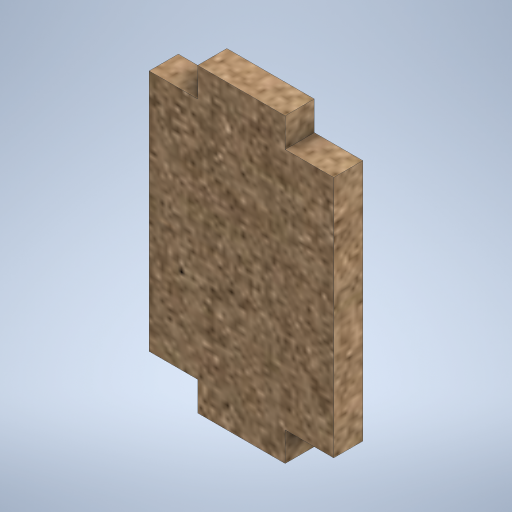
# Autodesk Inventor part: Wall_Base2
Saved by Autodesk Inventor 2024 (Build 280153000, 153)
## iProperties
Created: 2023-11-23
Part Number: Wall_Base2
Material: MDF Tablero de fibras de densidad media
Document SubType Name: Modeling
Designer: marco
Density: 0.8 g/cm^3
Appearance: Cartón - Ondulado
Author: marco
Autodesk Inventor part; units mm, degrees
ref_plane "YZ Plane" through (0, 0, 0) normal (1, 0, 0) x (0, 1, 0)
ref_plane "XZ Plane" through (0, 0, 0) normal (0, 1, 0) x (-1, 0, 0)
ref_plane "XY Plane" through (0, 0, 0) normal (0, 0, 1) x (1, 0, 0)
sketch "Boceto1" plane through (0, 0, 0) normal (0, 0, 1) x (1, 0, 0)
  line L0 (-4.5, 15.5) -> (-4.5, 12.5)
  line L1 (-4.5, 12.5) -> (-9.5, 12.5)
  line L2 (-9.5, 12.5) -> (-9.5, -12.5)
  line L3 (-9.5, -12.5) -> (-4.5, -12.5)
  line L4 (-4.5, -12.5) -> (-4.5, -15.5)
  line L5 (-4.5, -15.5) -> (-1.5, -15.5)
  line L6 (-1.5, 15.5) -> (-4.5, 15.5)
  line L7 (9.5, 12.5) -> (9.5, -12.5)
  line L8 (9.5, -12.5) -> (4.5, -12.5)
  line L9 (4.5, -12.5) -> (4.5, -15.5)
  line L10 (4.5, -15.5) -> (-4.5, -15.5)
  line L11 (-4.5, 15.5) -> (4.5, 15.5)
  line L12 (4.5, 15.5) -> (4.5, 12.5)
  line L13 (4.5, 12.5) -> (9.5, 12.5)
  constraints: 28 end point
extrude "Extrusión1" add sketch "Boceto1" along normal blind 3
